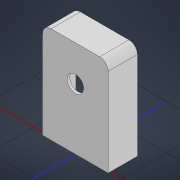
# Autodesk Inventor part: Camera-Cover
Saved by Autodesk Inventor 2022.2 (Build 262287010, 287A)
## iProperties
Created: 2022-04-02
Part Number: Camera-Cover
Material: Generisch
Document SubType Name: Modeling
Designer: sleib
Density: 1 g/cm^3
Appearance: Vorgabe
Author: sleib
Autodesk Inventor part; units mm, degrees
ref_plane "YZ Plane" through (0, 0, 0) normal (1, 0, 0) x (0, 1, 0)
ref_plane "XZ Plane" through (0, 0, 0) normal (0, 1, 0) x (-1, 0, 0)
ref_plane "XY Plane" through (0, 0, 0) normal (0, 0, 1) x (1, 0, 0)
sketch "Skizze1" plane through (0, 0, 0) normal (0, 0, 1) x (1, 0, 0)
  line L0 (-13, -20) -> (13, -20)
  line L1 (13, -20) -> (13, 18)
  line L2 (11, 20) -> (-11, 20)
  line L3 (-13, 18) -> (-13, -20)
  line L4 (-13, -20) -> (13, 20) construction
  line L5 (13, -20) -> (-13, 20) construction
  arc A0 (13, 18) -> (11, 20) centre (11, 18) ccw
  arc A1 (-11, 20) -> (-13, 18) centre (-11, 18) ccw
  line L6 (-11, 21.8) -> (11, 21.8)
  arc A2 (14.8, 18) -> (11, 21.8) centre (11, 18) ccw
  line L7 (14.8, 18) -> (14.8, -21.8)
  line L8 (14.8, -21.8) -> (-14.8, -21.8)
  line L9 (-14.8, -21.8) -> (-14.8, 18)
  arc A3 (-11, 21.8) -> (-14.8, 18) centre (-11, 18) ccw
  line L10 (-4.25, 10) -> (4.25, 10)
  line L11 (4.25, 10) -> (4.25, 1.5)
  line L12 (4.25, 1.5) -> (-4.25, 1.5)
  line L13 (-4.25, 1.5) -> (-4.25, 10)
  circle A4 centre (0, 5.75) radius 4.25 construction
  line L14 (0, 20) -> (0, -20) construction
  circle A5 centre (0, 5.75) radius 3.75
  point P0 (0, 0)
  dimension "d0" = 26
  dimension "d7" = 2
  dimension "d8" = 1.8
  dimension "d13" = 21.5
  dimension "d14" = 8.5
  dimension "d15" = 7.5
  dimension "d16" = 40
  constraints: 30 end point, 8 point on circle, 7 tangent, 6 centre point, 6 parallel, 5 point on line, 4 midpoint, 4 perpendicular, 2 horizontal, 1 coincident, 1 equal radius, 5 other
  measures "d0" distance of L5.end L4.end
  measures "d7" radius of A0
  measures "d8" distance between parallel lines of L2 L6
  measures "d13" distance between parallel lines of L12 L0
  measures "d14" distance of L12.end L10.start
  measures "d15" diameter of A5
  measures "d16" distance between parallel lines of L0 L2
extrude "Extrusion1" add sketch "Skizze1" against normal blind 12 contours L6 A2 L7 L8 L9 A3
extrude "Extrusion2" add sketch "Skizze1" along normal blind 1.2 contours L3 A1 L2 A0 L1 L0 | L6 A2 L7 L8 L9 A3 | L10 L11 L12 L13
sketch "Skizze2" plane through (-14.8, -21.8, -12) normal (0, -1, 0) x (1, 0, 0)
  line L0 (0, 0) -> (0, 13.2) projected
  line L1 (29.6, 0) -> (0, 0) projected
  line L2 (29.6, 0) -> (29.6, 13.2) projected
  line L3 (0, 13.2) -> (29.6, 13.2) projected
  line L4 (3.8, 0) -> (25.8, 0) projected
  line L5 (7.3, 0) -> (22.3, 0)
  line L6 (22.3, 0) -> (22.3, 7)
  line L7 (22.3, 7) -> (7.3, 7)
  line L8 (7.3, 7) -> (7.3, 0)
  point P0 (14.8, 12)
  point P1 (14.8, 0)
  point P2 (22.3, 0)
  dimension "d9" = 15
  dimension "d10" = 7
  constraints: 8 end point, 2 midpoint, 2 parallel, 1 horizontal, 1 perpendicular, 1 point on line
  measures "d9" distance between parallel lines of L6 L8
  measures "d10" distance of L5.end L6.end
extrude "Extrusion3" cut sketch "Skizze2" against normal up to next contours L8 L7 L6 L1
